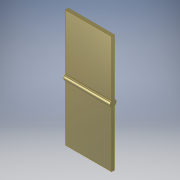
# Autodesk Inventor part: Flat Hinge
Saved by Autodesk Inventor 2018 (Build 220112000, 112)
## iProperties
Created: 2018-02-19
Part Number: Flat Hinge
Material: Generic
Document SubType Name: Modeling
Designer: Melda
Density: 1 g/cm^3
Appearance: Gold - Metal
Author: Melda
Autodesk Inventor part; units mm, degrees
ref_plane "YZ Plane" through (0, 0, 0) normal (1, 0, 0) x (0, 1, 0)
ref_plane "XZ Plane" through (0, 0, 0) normal (0, 1, 0) x (-1, 0, 0)
ref_plane "XY Plane" through (0, 0, 0) normal (0, 0, 1) x (1, 0, 0)
sketch "Sketch1" plane through (0, 0, 0) normal (1, 0, 0) x (0, 1, 0)
  line L0 (1.7321, 1) -> (37.9989, 1)
  line L1 (37.9989, 1) -> (37.9989, -1)
  line L2 (37.9989, -1) -> (1.7321, -1)
  line L3 (-1.7321, 1) -> (-37.9989, 1)
  line L4 (-37.9989, 1) -> (-37.9989, -1)
  line L5 (-37.9989, -1) -> (-1.7321, -1)
  arc A0 (1.7321, 1) -> (-1.7321, 1) centre (0, 0) ccw
  arc A1 (-1.7321, -1) -> (1.7321, -1) centre (0, 0) ccw
  dimension "d1" = 2
  constraints: 12 end point, 4 point on circle, 2 centre point, 1 coincident, 1 horizontal, 1 parallel, 1 perpendicular
  measures "d1" distance of L0.end L1.end
extrude "Extrusion1" add sketch "Sketch1" along normal blind 30
body "Solid1"
